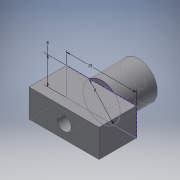
# Autodesk Inventor part: wierd bearing interface part
Saved by Autodesk Inventor 2019 (Build 230136000, 136)
## iProperties
Created: 2022-03-28
Part Number: wierd bearing interface part
Material: Generic
Document SubType Name: Modeling
Designer: Ian
Density: 1 g/cm^3
Appearance: Default
Author: Ian
Autodesk Inventor part; units mm, degrees
ref_plane "YZ Plane" through (0, 0, 0) normal (1, 0, 0) x (0, 1, 0)
ref_plane "XZ Plane" through (0, 0, 0) normal (0, 1, 0) x (-1, 0, 0)
ref_plane "XY Plane" through (0, 0, 0) normal (0, 0, 1) x (1, 0, 0)
sketch "Sketch1" plane through (0, 0, 0) normal (0, 0, 1) x (1, 0, 0)
  line L0 (-7.5, 3) -> (7.5, 3)
  line L1 (7.5, 3) -> (7.5, -3)
  line L2 (7.5, -3) -> (-7.5, -3)
  line L3 (-7.5, -3) -> (-7.5, 3)
  circle A0 centre (0, 0) radius 4
  line L4 (-7.5, 3) -> (7.5, -3) construction
  dimension "d0" = 6
  dimension "d1" = 15
  dimension "d2" = 8
  constraints: 10 end point, 2 coincident, 2 parallel, 1 centre point, 1 horizontal, 1 midpoint, 1 perpendicular
  measures "d0" distance of L2.end L0.start
  measures "d1" distance of L0.start L0.end
  measures "d2" diameter of A0
extrude "Extrusion1" add sketch "Sketch1" along normal blind 8 contours L0 A0 L2 L3 | L0 A0 L2 | L0 L1 L2 A0
extrude "Extrusion2" add sketch "Sketch1" against normal blind 8 contours A0 L0 | L0 A0 L2 | L2 A0
sketch "Sketch2" plane through (0, 0, 8) normal (0, 0, 1) x (1, 0, 0)
  circle A0 centre (0, 0) radius 1.5
  dimension "d7" = 3
  constraints: 1 centre point, 1 coincident
  measures "d7" diameter of A0
extrude "Extrusion3" cut sketch "Sketch2" against normal through all
sketch "Sketch3" plane through (-7.5, 3, 8) normal (0, 1, 0) x (1, 0, 0)
  circle A0 centre (3.75, 4) radius 1.5
  circle A1 centre (11.25, 4) radius 1.5
  line L0 (3.75, 4) -> (0, 4)
  line L1 (0, 8) -> (0, 0) projected
  line L2 (3.75, 4) -> (7.5, 4)
  line L3 (7.5, 4) -> (11.25, 4)
  line L4 (11.25, 4) -> (15, 4)
  line L5 (15, 8) -> (15, 0) projected
  point P0 (7.5, 8)
  dimension "d10" = 3
  dimension "d11" = 3
  constraints: 8 end point, 5 collinear, 2 centre point, 2 midpoint, 1 point on line
  measures "d10" diameter of A0
  measures "d11" diameter of A1
extrude "Extrusion4" cut sketch "Sketch3" against normal through all
sketch "Sketch4" plane through (0, 0, -8) normal (0, 0, -1) x (-1, 0, 0)
  circle A0 centre (0, 0) radius 2.5
  line L0 (1.5, -2) -> (-1.5, -2)
  dimension "d14" = 5
  dimension "d15" = 4.5
  constraints: 2 end point, 2 point on circle, 1 centre point, 1 coincident, 1 horizontal
  measures "d14" diameter of A0
extrude "Extrusion5" cut sketch "Sketch4" against normal blind 16.75 contours A0 L0 picked at (0.6276, -0.7851)
body "Solid1"
